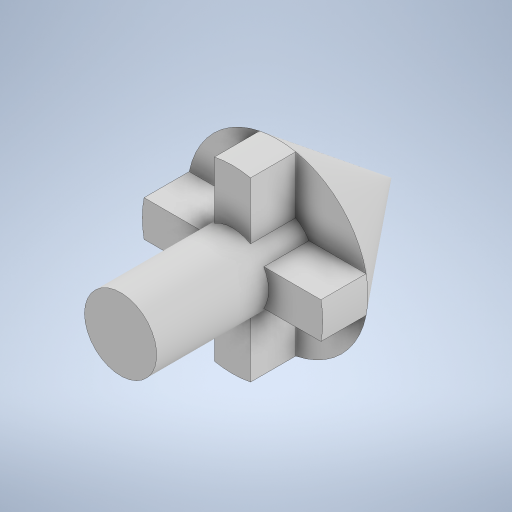
# Autodesk Inventor part: Goma tacómetro
Saved by Autodesk Inventor 2023 (Build 270158000, 158)
## iProperties
Created: 2023-07-25
Part Number: Goma tacómetro
Material: Generic
Document SubType Name: Modeling
Designer: romy_
Density: 1 g/cm^3
Appearance: Default
Author: romy_
Autodesk Inventor part; units mm, degrees
ref_plane "YZ Plane" through (0, 0, 0) normal (1, 0, 0) x (0, 1, 0)
ref_plane "XZ Plane" through (0, 0, 0) normal (0, 1, 0) x (-1, 0, 0)
ref_plane "XY Plane" through (0, 0, 0) normal (0, 0, 1) x (1, 0, 0)
sketch "Sketch1" plane through (0, 0, 0) normal (0, 1, 0) x (-1, 0, 0)
  line L0 (0, 0) -> (2, 0)
  line L1 (2, 0) -> (2, -8.7)
  line L2 (2, -8.7) -> (5, -8.7)
  line L3 (5, -8.7) -> (0, -15)
  line L4 (0, -15) -> (0, 0)
  dimension "d0" = 15
  dimension "d1" = 5
  dimension "d3" = 2
  dimension "d5" = 8.7
  constraints: 10 end point, 2 horizontal, 2 vertical
  measures "d0" distance of L3.end L0.start
  measures "d1" distance from line of L4 L2.end
  measures "d3" distance from line of L4 L1.end
  measures "d5" distance from line of L0 L2.end
revolve "Revolution1" add sketch "Sketch1" angle 360 about axis through (0, 0, -15) along (0, 0, 1)
sketch "Sketch2" plane through (0, 0, -8.7) normal (0, 0, 1) x (1, 0, 0)
  circle A0 centre (0, 0) radius 2 projected
  circle A1 centre (0, 0) radius 5 projected
  line L0 (1.7321, 1) -> (4.899, 1)
  line L1 (0, 0) -> (5, 0) construction
  line L2 (1.7321, -1) -> (4.899, -1)
  line L3 (-1, 1.7321) -> (-1, 4.899)
  line L4 (1, 1.7321) -> (1, 4.899)
  line L5 (-1.7321, -1) -> (-4.899, -1)
  line L6 (-1.7321, 1) -> (-4.899, 1)
  line L7 (1, -1.7321) -> (1, -4.899)
  line L8 (-1, -1.7321) -> (-1, -4.899)
  dimension "d8" = 1
  dimension "d11" = 360
  constraints: 18 end point, 2 horizontal, 2 point on circle, 2 symmetric about line, 27 other
  measures "d8" distance from line of point (0, 0) L0
extrude "Extrusion1" add sketch "Sketch2" along normal blind 2.5 contours A0 L0 A1 L2 | A0 L3 A1 L4 | L7 A1 L8 A0 | A0 L5 A1 L6
body "Solid1"
